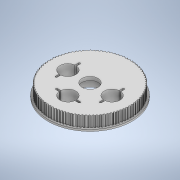
# Autodesk Inventor part: os_6_zebatka
Saved by Autodesk Inventor 2020.3 (Build 243373000, 373)
## iProperties
Created: 2021-03-12
Part Number: os_6_zebatka
Material: Generic
Document SubType Name: Modeling
Designer: patry
Density: 1 g/cm^3
Appearance: Default
Author: patry
Autodesk Inventor part; units mm, degrees
(part 1 of 2)
ref_plane "YZ Plane" through (0, 0, 0) normal (1, 0, 0) x (0, 1, 0)
ref_plane "XZ Plane" through (0, 0, 0) normal (0, 1, 0) x (-1, 0, 0)
ref_plane "XY Plane" through (0, 0, 0) normal (0, 0, 1) x (1, 0, 0)
sketch "Sketch1" plane through (0, 0, 0) normal (0, 1, 0) x (-1, 0, 0)
  circle A0 centre (0, 0) radius 47.5
  dimension "d0" = 95
  constraints: 1 centre point, 1 coincident
  measures "d0" diameter of A0
extrude "Extrusion1" add sketch "Sketch1" along normal blind 2
sketch "Sketch2" plane through (0, 2, 0) normal (0, 1, 0) x (1, 0, 0)
  circle A0 centre (0, 0) radius 45.5
  line L0 (0, 45.5) -> (0.3625, 45.5)
  line L1 (0.3625, 45.5) -> (-0.3625, 45.5)
  line L2 (-0.3625, 45.5) -> (0.3625, 45.5)
  arc A1 (-1.5, 44.3625) -> (-0.5625, 45.3) centre (-1.5, 45.3) ccw
  arc A2 (0.5625, 45.3) -> (1.5, 44.3625) centre (1.5, 45.3) ccw
  line L3 (-0.3625, 45.5) -> (0.3625, 45.5)
  arc A3 (-0.3625, 45.5) -> (-0.5625, 45.3) centre (-0.3625, 45.3) ccw
  arc A4 (0.5625, 45.3) -> (0.3625, 45.5) centre (0.3625, 45.3) ccw
  line L4 (-2.9452, 45.4046) -> (-2.5835, 45.428)
  line L5 (-2.5835, 45.428) -> (-3.3069, 45.3811)
  line L6 (-3.3069, 45.3811) -> (-2.5835, 45.428)
  arc A5 (-4.3684, 44.1724) -> (-3.4936, 45.1686) centre (-4.4291, 45.1079) ccw
  arc A6 (-2.3709, 45.2414) -> (-1.3747, 44.3666) centre (-1.4354, 45.3021) ccw
  line L7 (-3.3069, 45.3811) -> (-2.5835, 45.428)
  arc A7 (-3.3069, 45.3811) -> (-3.4936, 45.1686) centre (-3.294, 45.1815) ccw
  arc A8 (-2.3709, 45.2414) -> (-2.5835, 45.428) centre (-2.5705, 45.2285) ccw
  line L8 (-5.8781, 45.1187) -> (-5.5186, 45.1655)
  line L9 (-5.5186, 45.1655) -> (-6.2375, 45.0719)
  line L10 (-6.2375, 45.0719) -> (-5.5186, 45.1655)
  arc A9 (-7.2185, 43.797) -> (-6.41, 44.8477) centre (-7.3397, 44.7266) ccw
  arc A10 (-5.2944, 44.9931) -> (-4.2437, 44.1845) centre (-4.3648, 45.1142) ccw
  line L11 (-6.2375, 45.0719) -> (-5.5186, 45.1655)
  arc A11 (-6.2375, 45.0719) -> (-6.41, 44.8477) centre (-6.2117, 44.8736) ccw
  arc A12 (-5.2944, 44.9931) -> (-5.5186, 45.1655) centre (-5.4928, 44.9672) ccw
  line L12 (-8.7863, 44.6436) -> (-8.4306, 44.7136)
  line L13 (-8.4306, 44.7136) -> (-9.1419, 44.5736)
  line L14 (-9.1419, 44.5736) -> (-8.4306, 44.7136)
  arc A13 (-10.0384, 43.2379) -> (-9.2996, 44.3388) centre (-10.2194, 44.1577) ccw
  arc A14 (-8.1957, 44.556) -> (-7.0948, 43.8172) centre (-7.2759, 44.737) ccw
  line L15 (-9.1419, 44.5736) -> (-8.4306, 44.7136)
  arc A15 (-9.1419, 44.5736) -> (-9.2996, 44.3388) centre (-9.1033, 44.3774) ccw
  arc A16 (-8.1957, 44.556) -> (-8.4306, 44.7136) centre (-8.392, 44.5174) ccw
  line L16 (-11.6576, 43.9812) -> (-11.3072, 44.0741)
  line L17 (-11.3072, 44.0741) -> (-12.008, 43.8884)
  line L18 (-12.008, 43.8884) -> (-11.3072, 44.0741)
  arc A17 (-12.8161, 42.4974) -> (-12.1501, 43.6438) centre (-13.0563, 43.4036) ccw
  arc A18 (-11.0626, 43.932) -> (-9.9162, 43.266) centre (-10.1564, 44.1722) ccw
  line L19 (-12.008, 43.8884) -> (-11.3072, 44.0741)
  arc A19 (-12.008, 43.8884) -> (-12.1501, 43.6438) centre (-11.9568, 43.695) ccw
  arc A20 (-11.0626, 43.932) -> (-11.3072, 44.0741) centre (-11.256, 43.8808) ccw
  line L20 (-14.4801, 43.1344) -> (-14.1364, 43.2498)
  line L21 (-14.1364, 43.2498) -> (-14.8237, 43.0191)
  line L22 (-14.8237, 43.0191) -> (-14.1364, 43.2498)
  arc A21 (-15.5401, 41.5787) -> (-14.9497, 42.7658) centre (-15.8384, 42.4675) ccw
  arc A22 (-13.8832, 43.1238) -> (-12.696, 42.5334) centre (-12.9944, 43.4222) ccw
  line L23 (-14.8237, 43.0191) -> (-14.1364, 43.2498)
  arc A23 (-14.8237, 43.0191) -> (-14.9497, 42.7658) centre (-14.7601, 42.8295) ccw
  arc A24 (-13.8832, 43.1238) -> (-14.1364, 43.2498) centre (-14.0728, 43.0602) ccw
  line L24 (-17.2418, 42.1067) -> (-16.9063, 42.244)
  line L25 (-16.9063, 42.244) -> (-17.5772, 41.9693)
  line L26 (-17.5772, 41.9693) -> (-16.9063, 42.244)
  arc A25 (-18.1989, 40.4856) -> (-17.6865, 41.7084) centre (-18.5541, 41.3532) ccw
  arc A26 (-16.6454, 42.1347) -> (-15.4226, 41.6224) centre (-15.7779, 42.49) ccw
  line L27 (-17.5772, 41.9693) -> (-16.9063, 42.244)
  arc A27 (-17.5772, 41.9693) -> (-17.6865, 41.7084) centre (-17.5014, 41.7842) ccw
  arc A28 (-16.6454, 42.1347) -> (-16.9063, 42.244) centre (-16.8305, 42.0589) ccw
  line L28 (-19.9312, 40.9023) -> (-19.6053, 41.0611)
  line L29 (-19.6053, 41.0611) -> (-20.257, 40.7435)
  line L30 (-20.257, 40.7435) -> (-19.6053, 41.0611)
  arc A29 (-20.7813, 39.2227) -> (-20.3492, 40.4761) centre (-21.192, 40.0654) ccw
  arc A30 (-19.3379, 40.9689) -> (-18.0845, 40.5368) centre (-18.4951, 41.3796) ccw
  line L31 (-20.257, 40.7435) -> (-19.6053, 41.0611)
  arc A31 (-20.257, 40.7435) -> (-20.3492, 40.4761) centre (-20.1694, 40.5637) ccw
  arc A32 (-19.3379, 40.9689) -> (-19.6053, 41.0611) centre (-19.5177, 40.8813) ccw
  line L32 (-22.537, 39.5264) -> (-22.2221, 39.7059)
  line L33 (-22.2221, 39.7059) -> (-22.8519, 39.3468)
  line L34 (-22.8519, 39.3468) -> (-22.2221, 39.7059)
  arc A33 (-23.2766, 37.7952) -> (-22.9266, 39.074) centre (-23.741, 38.6097) ccw
  arc A34 (-21.9493, 39.6313) -> (-20.6705, 39.2812) centre (-21.1348, 40.0956) ccw
  line L35 (-22.8519, 39.3468) -> (-22.2221, 39.7059)
  arc A35 (-22.8519, 39.3468) -> (-22.9266, 39.074) centre (-22.7528, 39.1731) ccw
  arc A36 (-21.9493, 39.6313) -> (-22.2221, 39.7059) centre (-22.123, 39.5322) ccw
  line L36 (-25.0482, 37.9847) -> (-24.7456, 38.1842)
  line L37 (-24.7456, 38.1842) -> (-25.3509, 37.7851)
  line L38 (-25.3509, 37.7851) -> (-24.7456, 38.1842)
  arc A37 (-25.6743, 36.2093) -> (-25.4077, 37.508) centre (-26.1904, 36.9919) ccw
  arc A38 (-24.4685, 38.1274) -> (-23.1698, 37.8608) centre (-23.6859, 38.6435) ccw
  line L39 (-25.3509, 37.7851) -> (-24.7456, 38.1842)
  arc A39 (-25.3509, 37.7851) -> (-25.4077, 37.508) centre (-25.2408, 37.6182) ccw
  arc A40 (-24.4685, 38.1274) -> (-24.7456, 38.1842) centre (-24.6355, 38.0173) ccw
  line L40 (-27.4545, 36.2836) -> (-27.1654, 36.5024)
  line L41 (-27.1654, 36.5024) -> (-27.7435, 36.0649)
  line L42 (-27.7435, 36.0649) -> (-27.1654, 36.5024)
  arc A41 (-27.9643, 34.4715) -> (-27.7823, 35.7847) centre (-28.5299, 35.2191) ccw
  arc A42 (-26.8852, 36.4636) -> (-25.5719, 36.2816) centre (-26.1376, 37.0293) ccw
  line L43 (-27.7435, 36.0649) -> (-27.1654, 36.5024)
  arc A43 (-27.7435, 36.0649) -> (-27.7823, 35.7847) centre (-27.6228, 35.9054) ccw
  arc A44 (-26.8852, 36.4636) -> (-27.1654, 36.5024) centre (-27.0447, 36.3429) ccw
  line L44 (-29.7455, 34.4304) -> (-29.4712, 34.6674)
  line L45 (-29.4712, 34.6674) -> (-30.0198, 34.1934)
  line L46 (-30.0198, 34.1934) -> (-29.4712, 34.6674)
  arc A45 (-30.1369, 32.5891) -> (-30.0404, 33.9114) centre (-30.7498, 33.2985) ccw
  arc A46 (-29.1891, 34.6468) -> (-27.8668, 34.5503) centre (-28.4797, 35.2597) ccw
  line L47 (-30.0198, 34.1934) -> (-29.4712, 34.6674)
  arc A47 (-30.0198, 34.1934) -> (-30.0404, 33.9114) centre (-29.8891, 34.0421) ccw
  arc A48 (-29.1891, 34.6468) -> (-29.4712, 34.6674) centre (-29.3405, 34.5161) ccw
  line L48 (-31.9118, 32.4328) -> (-31.6534, 32.687)
  line L49 (-31.6534, 32.687) -> (-32.1702, 32.1786)
  line L50 (-32.1702, 32.1786) -> (-31.6534, 32.687)
  arc A49 (-32.1832, 30.5699) -> (-32.1725, 31.8957) centre (-32.8407, 31.2382) ccw
  arc A50 (-31.3706, 32.6848) -> (-30.0448, 32.674) centre (-30.7023, 33.3423) ccw
  line L51 (-32.1702, 32.1786) -> (-31.6534, 32.687)
  arc A51 (-32.1702, 32.1786) -> (-32.1725, 31.8957) centre (-32.0299, 32.036) ccw
  arc A52 (-31.3706, 32.6848) -> (-31.6534, 32.687) centre (-31.5131, 32.5445) ccw
  line L52 (-33.9442, 30.2991) -> (-33.7029, 30.5696)
  line L53 (-33.7029, 30.5696) -> (-34.1856, 30.0287)
  line L54 (-34.1856, 30.0287) -> (-33.7029, 30.5696)
  arc A53 (-34.0945, 28.4226) -> (-34.1696, 29.7463) centre (-34.7939, 29.0469) ccw
  arc A54 (-33.4205, 30.5856) -> (-32.0968, 30.6607) centre (-32.7962, 31.285) ccw
  line L55 (-34.1856, 30.0287) -> (-33.7029, 30.5696)
  arc A55 (-34.1856, 30.0287) -> (-34.1696, 29.7463) centre (-34.0364, 29.8955) ccw
  arc A56 (-33.4205, 30.5856) -> (-33.7029, 30.5696) centre (-33.5536, 30.4364) ccw
  line L56 (-35.8343, 28.0384) -> (-35.6109, 28.3239)
  line L57 (-35.6109, 28.3239) -> (-36.0577, 27.7529)
  line L58 (-36.0577, 27.7529) -> (-35.6109, 28.3239)
  arc A57 (-35.8628, 26.1561) -> (-36.0234, 27.4721) centre (-36.6011, 26.7338) ccw
  arc A58 (-35.3302, 28.3582) -> (-34.0141, 28.5188) centre (-34.7525, 29.0965) ccw
  line L59 (-36.0577, 27.7529) -> (-35.6109, 28.3239)
  arc A59 (-36.0577, 27.7529) -> (-36.0234, 27.4721) centre (-35.9002, 27.6297) ccw
  arc A60 (-35.3302, 28.3582) -> (-35.6109, 28.3239) centre (-35.4534, 28.2006) ccw
  line L60 (-37.5741, 25.66) -> (-37.3697, 25.9594)
  line L61 (-37.3697, 25.9594) -> (-37.7785, 25.3607)
  line L62 (-37.7785, 25.3607) -> (-37.3697, 25.9594)
  arc A61 (-37.4807, 23.7798) -> (-37.7262, 25.0827) centre (-38.2549, 24.3085) ccw
  arc A62 (-37.0917, 26.0118) -> (-35.7888, 26.2572) centre (-36.563, 26.786) ccw
  line L63 (-37.7785, 25.3607) -> (-37.3697, 25.9594)
  arc A63 (-37.7785, 25.3607) -> (-37.7262, 25.0827) centre (-37.6134, 25.2479) ccw
  arc A64 (-37.0917, 26.0118) -> (-37.3697, 25.9594) centre (-37.2045, 25.8466) ccw
  line L64 (-39.1563, 23.1741) -> (-38.9716, 23.486)
  line L65 (-38.9716, 23.486) -> (-39.3409, 22.8621)
  line L66 (-39.3409, 22.8621) -> (-38.9716, 23.486)
  arc A65 (-38.9413, 21.3039) -> (-39.2706, 22.5881) centre (-39.7481, 21.7813) ccw
  arc A66 (-38.6977, 23.5563) -> (-37.4134, 23.8856) centre (-38.2202, 24.3631) ccw
  line L67 (-39.3409, 22.8621) -> (-38.9716, 23.486)
  arc A67 (-39.3409, 22.8621) -> (-39.2706, 22.5881) centre (-39.1688, 22.7602) ccw
  arc A68 (-38.6977, 23.5563) -> (-38.9716, 23.486) centre (-38.7995, 23.3842) ccw
  line L68 (-40.5742, 20.5909) -> (-40.4101, 20.9141)
  line L69 (-40.4101, 20.9141) -> (-40.7382, 20.2676)
  line L70 (-40.7382, 20.2676) -> (-40.4101, 20.9141)
  arc A69 (-40.2387, 18.7385) -> (-40.6504, 19.9988) centre (-41.0747, 19.1628) ccw
  arc A70 (-40.1413, 21.002) -> (-38.881, 21.4137) centre (-39.717, 21.838) ccw
  line L71 (-40.7382, 20.2676) -> (-40.4101, 20.9141)
  arc A71 (-40.7382, 20.2676) -> (-40.6504, 19.9988) centre (-40.5599, 20.1771) ccw
  arc A72 (-40.1413, 21.002) -> (-40.4101, 20.9141) centre (-40.2318, 20.8236) ccw
  line L72 (-41.8219, 17.9213) -> (-41.6792, 18.2545)
  line L73 (-41.6792, 18.2545) -> (-41.9647, 17.5882)
  line L74 (-41.9647, 17.5882) -> (-41.6792, 18.2545)
  arc A73 (-41.3672, 16.0946) -> (-41.8597, 17.3255) centre (-42.2289, 16.4638) ccw
  arc A74 (-41.4166, 18.3596) -> (-40.1856, 18.8521) centre (-41.0473, 19.2213) ccw
  line L75 (-41.9647, 17.5882) -> (-41.6792, 18.2545)
  arc A75 (-41.9647, 17.5882) -> (-41.8597, 17.3255) centre (-41.7809, 17.5094) ccw
  arc A76 (-41.4166, 18.3596) -> (-41.6792, 18.2545) centre (-41.4953, 18.1758) ccw
  line L76 (-42.8943, 15.1766) -> (-42.7734, 15.5184)
  line L77 (-42.7734, 15.5184) -> (-43.0152, 14.8349)
  line L78 (-43.0152, 14.8349) -> (-42.7734, 15.5184)
  arc A77 (-42.3223, 13.3831) -> (-42.8934, 14.5796) centre (-43.2061, 13.6958) ccw
  arc A78 (-42.5181, 15.6402) -> (-41.3216, 16.2113) centre (-42.2054, 16.524) ccw
  line L79 (-43.0152, 14.8349) -> (-42.7734, 15.5184)
  arc A79 (-43.0152, 14.8349) -> (-42.8934, 14.5796) centre (-42.8267, 14.7682) ccw
  arc A80 (-42.5181, 15.6402) -> (-42.7734, 15.5184) centre (-42.5848, 15.4517) ccw
  line L80 (-43.7867, 12.3683) -> (-43.6882, 12.7171)
  line L81 (-43.6882, 12.7171) -> (-43.8852, 12.0194)
  line L82 (-43.8852, 12.0194) -> (-43.6882, 12.7171)
  arc A81 (-43.0998, 10.6155) -> (-43.7471, 11.7726) centre (-44.002, 10.8704) ccw
  arc A82 (-43.4413, 12.8552) -> (-42.2843, 13.5026) centre (-43.1865, 13.7574) ccw
  line L83 (-43.8852, 12.0194) -> (-43.6882, 12.7171)
  arc A83 (-43.8852, 12.0194) -> (-43.7471, 11.7726) centre (-43.6928, 11.9651) ccw
  arc A84 (-43.4413, 12.8552) -> (-43.6882, 12.7171) centre (-43.4957, 12.6628) ccw
  line L84 (-44.4955, 9.508) -> (-44.4197, 9.8625)
  line L85 (-44.4197, 9.8625) -> (-44.5712, 9.1535)
  line L86 (-44.5712, 9.1535) -> (-44.4197, 9.8625)
  arc A85 (-43.6965, 7.8034) -> (-44.4174, 8.9161) centre (-44.6133, 7.9993) ccw
  arc A86 (-44.1823, 10.0163) -> (-43.0696, 10.7372) centre (-43.9864, 10.9331) ccw
  line L87 (-44.5712, 9.1535) -> (-44.4197, 9.8625)
  arc A87 (-44.5712, 9.1535) -> (-44.4174, 8.9161) centre (-44.3756, 9.1117) ccw
  arc A88 (-44.1823, 10.0163) -> (-44.4197, 9.8625) centre (-44.2241, 9.8207) ccw
  line L88 (-45.0176, 6.6079) -> (-44.965, 6.9666)
  line L89 (-44.965, 6.9666) -> (-45.0703, 6.2492)
  line L90 (-45.0703, 6.2492) -> (-44.965, 6.9666)
  arc A89 (-44.11, 4.9586) -> (-44.9014, 6.0223) centre (-45.0376, 5.0948) ccw
  arc A90 (-44.738, 7.1354) -> (-43.6743, 7.9268) centre (-44.6019, 8.063) ccw
  line L91 (-45.0703, 6.2492) -> (-44.965, 6.9666)
  arc A91 (-45.0703, 6.2492) -> (-44.9014, 6.0223) centre (-44.8724, 6.2202) ccw
  arc A92 (-44.738, 7.1354) -> (-44.965, 6.9666) centre (-44.7671, 6.9375) ccw
  line L92 (-45.3509, 3.6801) -> (-45.3216, 4.0414)
  line L93 (-45.3216, 4.0414) -> (-45.3803, 3.3187)
  line L94 (-45.3803, 3.3187) -> (-45.3216, 4.0414)
  arc A93 (-44.3385, 2.093) -> (-45.1971, 3.1032) centre (-45.2729, 2.1688) ccw
  arc A94 (-45.1061, 4.2245) -> (-44.0958, 5.0831) centre (-45.0303, 5.159) ccw
  line L95 (-45.3803, 3.3187) -> (-45.3216, 4.0414)
  arc A95 (-45.3803, 3.3187) -> (-45.1971, 3.1032) centre (-45.1809, 3.3026) ccw
  arc A96 (-45.1061, 4.2245) -> (-45.3216, 4.0414) centre (-45.1223, 4.0252) ccw
  line L96 (-45.494, 0.7368) -> (-45.4882, 1.0992)
  line L97 (-45.4882, 1.0992) -> (-45.4999, 0.3743)
  line L98 (-45.4999, 0.3743) -> (-45.4882, 1.0992)
  arc A97 (-44.381, -0.7814) -> (-45.3032, 0.1711) centre (-45.3184, -0.7663) ccw
  arc A98 (-45.285, 1.296) -> (-44.3324, 2.2182) centre (-45.2698, 2.2333) ccw
  line L99 (-45.4999, 0.3743) -> (-45.4882, 1.0992)
  arc A99 (-45.4999, 0.3743) -> (-45.3032, 0.1711) centre (-45.2999, 0.3711) ccw
  arc A100 (-45.285, 1.296) -> (-45.4882, 1.0992) centre (-45.2882, 1.096) ccw
  line L100 (-45.4463, -2.2096) -> (-45.4639, -1.8475)
  line L101 (-45.4639, -1.8475) -> (-45.4287, -2.5717)
  line L102 (-45.4287, -2.5717) -> (-45.4639, -1.8475)
  arc A101 (-44.2373, -3.6526) -> (-45.2192, -2.7617) centre (-45.1737, -3.6981) ccw
  arc A102 (-45.2739, -1.638) -> (-44.383, -0.6561) centre (-45.3194, -0.7016) ccw
  line L103 (-45.4287, -2.5717) -> (-45.4639, -1.8475)
  arc A103 (-45.4287, -2.5717) -> (-45.2192, -2.7617) centre (-45.2289, -2.5619) ccw
  arc A104 (-45.2739, -1.638) -> (-45.4639, -1.8475) centre (-45.2642, -1.8378) ccw
  line L104 (-45.208, -5.1467) -> (-45.249, -4.7865)
  line L105 (-45.249, -4.7865) -> (-45.167, -5.5069)
  line L106 (-45.167, -5.5069) -> (-45.249, -4.7865)
  arc A105 (-43.9081, -6.5084) -> (-44.9456, -5.6829) centre (-44.8396, -6.6144) ccw
  arc A106 (-45.0729, -4.5652) -> (-44.2475, -3.5276) centre (-45.1789, -3.6337) ccw
  line L107 (-45.167, -5.5069) -> (-45.249, -4.7865)
  arc A107 (-45.167, -5.5069) -> (-44.9456, -5.6829) centre (-44.9683, -5.4842) ccw
  arc A108 (-45.0729, -4.5652) -> (-45.249, -4.7865) centre (-45.0503, -4.7639) ccw
  line L108 (-44.78, -8.0622) -> (-44.8443, -7.7054)
  line L109 (-44.8443, -7.7054) -> (-44.7158, -8.419)
  line L110 (-44.7158, -8.419) -> (-44.8443, -7.7054)
  arc A109 (-43.3947, -9.3369) -> (-44.4835, -8.5804) centre (-44.3174, -9.503) ccw
  arc A110 (-44.6829, -7.4732) -> (-43.9263, -6.3844) centre (-44.849, -6.5505) ccw
  line L111 (-44.7158, -8.419) -> (-44.8443, -7.7054)
  arc A111 (-44.7158, -8.419) -> (-44.4835, -8.5804) centre (-44.519, -8.3835) ccw
  arc A112 (-44.6829, -7.4732) -> (-44.8443, -7.7054) centre (-44.6474, -7.67) ccw
  line L112 (-44.1643, -10.9439) -> (-44.2514, -10.592)
  line L113 (-44.2514, -10.592) -> (-44.0771, -11.2957)
  line L114 (-44.0771, -11.2957) -> (-44.2514, -10.592)
  arc A113 (-42.6994, -12.1263) -> (-43.8348, -11.4418) centre (-43.6093, -12.3517) ccw
  arc A114 (-44.1054, -10.3498) -> (-43.4209, -9.2143) centre (-44.3309, -9.4398) ccw
  line L115 (-44.0771, -11.2957) -> (-44.2514, -10.592)
  arc A115 (-44.0771, -11.2957) -> (-43.8348, -11.4418) centre (-43.8829, -11.2476) ccw
  arc A116 (-44.1054, -10.3498) -> (-44.2514, -10.592) centre (-44.0573, -10.5439) ccw
  line L116 (-43.3632, -13.7797) -> (-43.473, -13.4342)
  line L117 (-43.473, -13.4342) -> (-43.2535, -14.1252)
  line L118 (-43.2535, -14.1252) -> (-43.473, -13.4342)
  arc A117 (-41.8249, -14.8647) -> (-43.0023, -14.2552) centre (-42.7184, -15.1487) ccw
  arc A118 (-43.343, -13.183) -> (-42.7334, -12.0056) centre (-43.6269, -12.2896) ccw
  line L119 (-43.2535, -14.1252) -> (-43.473, -13.4342)
  arc A119 (-43.2535, -14.1252) -> (-43.0023, -14.2552) centre (-43.0628, -14.0646) ccw
  arc A120 (-43.343, -13.183) -> (-43.473, -13.4342) centre (-43.2824, -13.3736) ccw
  line L120 (-42.3803, -16.5577) -> (-42.5123, -16.22)
  line L121 (-42.5123, -16.22) -> (-42.2484, -16.8953)
  line L122 (-42.2484, -16.8953) -> (-42.5123, -16.22)
  arc A121 (-40.775, -17.5409) -> (-41.9894, -17.0088) centre (-41.6482, -17.882) ccw
  arc A122 (-42.3988, -15.961) -> (-41.8667, -14.7466) centre (-42.7399, -15.0877) ccw
  line L123 (-42.2484, -16.8953) -> (-42.5123, -16.22)
  arc A123 (-42.2484, -16.8953) -> (-41.9894, -17.0088) centre (-42.0621, -16.8225) ccw
  arc A124 (-42.3988, -15.961) -> (-42.5123, -16.22) centre (-42.326, -16.1472) ccw
  line L124 (-41.2197, -19.2662) -> (-41.3732, -18.9378)
  line L125 (-41.3732, -18.9378) -> (-41.0662, -19.5946)
  line L126 (-41.0662, -19.5946) -> (-41.3732, -18.9378)
  arc A125 (-39.554, -20.1435) -> (-40.8003, -19.6911) centre (-40.4034, -20.5404) ccw
  arc A126 (-41.2767, -18.672) -> (-40.8243, -17.4257) centre (-41.6737, -17.8226) ccw
  line L127 (-41.0662, -19.5946) -> (-41.3732, -18.9378)
  arc A127 (-41.0662, -19.5946) -> (-40.8003, -19.6911) centre (-40.885, -19.5099) ccw
  arc A128 (-41.2767, -18.672) -> (-41.3732, -18.9378) centre (-41.192, -18.8531) ccw
  line L128 (-39.8861, -21.894) -> (-40.0606, -21.5762)
  line L129 (-40.0606, -21.5762) -> (-39.7117, -22.2117)
  line L130 (-39.7117, -22.2117) -> (-40.0606, -21.5762)
  arc A129 (-38.1672, -22.6615) -> (-39.4402, -22.2908) centre (-38.989, -23.1127) ccw
  arc A130 (-39.9815, -21.3046) -> (-39.6108, -20.0317) centre (-40.4326, -20.4828) ccw
  line L131 (-39.7117, -22.2117) -> (-40.0606, -21.5762)
  arc A131 (-39.7117, -22.2117) -> (-39.4402, -22.2908) centre (-39.5364, -22.1155) ccw
  arc A132 (-39.9815, -21.3046) -> (-40.0606, -21.5762) centre (-39.8853, -21.4799) ccw
  line L132 (-38.3853, -24.4299) -> (-38.5799, -24.1241)
  line L133 (-38.5799, -24.1241) -> (-38.1907, -24.7357)
  line L134 (-38.1907, -24.7357) -> (-38.5799, -24.1241)
  arc A133 (-36.6203, -25.0846) -> (-37.9146, -24.797) centre (-37.4112, -25.5879) ccw
  arc A134 (-38.5186, -23.8479) -> (-38.2311, -22.5537) centre (-39.022, -23.057) ccw
  line L135 (-38.1907, -24.7357) -> (-38.5799, -24.1241)
  arc A135 (-38.1907, -24.7357) -> (-37.9146, -24.797) centre (-38.0219, -24.6283) ccw
  arc A136 (-38.5186, -23.8479) -> (-38.5799, -24.1241) centre (-38.4112, -24.0167) ccw
  line L136 (-36.7235, -26.8633) -> (-36.9375, -26.5707)
  line L137 (-36.9375, -26.5707) -> (-36.5094, -27.1559)
  line L138 (-36.5094, -27.1559) -> (-36.9375, -26.5707)
  arc A137 (-34.9198, -27.4024) -> (-36.2299, -27.1992) centre (-35.6764, -27.9559) ccw
  arc A138 (-36.8941, -26.2912) -> (-36.691, -24.9811) centre (-37.4476, -25.5346) ccw
  line L139 (-36.5094, -27.1559) -> (-36.9375, -26.5707)
  arc A139 (-36.5094, -27.1559) -> (-36.2299, -27.1992) centre (-36.348, -27.0378) ccw
  arc A140 (-36.8941, -26.2912) -> (-36.9375, -26.5707) centre (-36.7761, -26.4527) ccw
  line L140 (-34.9076, -29.1841) -> (-35.1401, -28.906)
  line L141 (-35.1401, -28.906) -> (-34.6751, -29.4622)
  line L142 (-34.6751, -29.4622) -> (-35.1401, -28.906)
  arc A141 (-33.0728, -29.6053) -> (-34.3934, -29.4873) centre (-33.792, -30.2066) ccw
  arc A142 (-35.1149, -28.6242) -> (-34.997, -27.3037) centre (-35.7163, -27.905) ccw
  line L143 (-34.6751, -29.4622) -> (-35.1401, -28.906)
  arc A143 (-34.6751, -29.4622) -> (-34.3934, -29.4873) centre (-34.5216, -29.3339) ccw
  arc A144 (-35.1149, -28.6242) -> (-35.1401, -28.906) centre (-34.9867, -28.7777) ccw
  line L144 (-32.9453, -31.3824) -> (-33.1953, -31.12)
  line L145 (-33.1953, -31.12) -> (-32.6953, -31.6449)
  line L146 (-32.6953, -31.6449) -> (-33.1953, -31.12)
  arc A145 (-31.0871, -31.684) -> (-32.4125, -31.6518) centre (-31.7659, -32.3306) ccw
  arc A146 (-33.1885, -30.8372) -> (-33.1563, -29.5118) centre (-33.8351, -30.1584) ccw
  line L147 (-32.6953, -31.6449) -> (-33.1953, -31.12)
  arc A147 (-32.6953, -31.6449) -> (-32.4125, -31.6518) centre (-32.5505, -31.507) ccw
  arc A148 (-33.1885, -30.8372) -> (-33.1953, -31.12) centre (-33.0505, -30.982) ccw
  line L148 (-30.8448, -33.4492) -> (-31.1113, -33.2034)
  line L149 (-31.1113, -33.2034) -> (-30.5783, -33.6949)
  line L150 (-30.5783, -33.6949) -> (-31.1113, -33.2034)
  arc A149 (-28.971, -33.6298) -> (-30.2957, -33.6835) centre (-29.6065, -34.319) ccw
  arc A150 (-31.1228, -32.9208) -> (-31.1764, -31.5961) centre (-31.812, -32.2853) ccw
  line L151 (-30.5783, -33.6949) -> (-31.1113, -33.2034)
  arc A151 (-30.5783, -33.6949) -> (-30.2957, -33.6835) centre (-30.4428, -33.5479) ccw
  arc A152 (-31.1228, -32.9208) -> (-31.1113, -33.2034) centre (-30.9757, -33.0564) ccw
  line L152 (-28.615, -35.3756) -> (-28.8968, -35.1476)
  line L153 (-28.8968, -35.1476) -> (-28.3331, -35.6036)
  line L154 (-28.3331, -35.6036) -> (-28.8968, -35.1476)
  arc A153 (-26.7334, -35.4346) -> (-28.0519, -35.5739) centre (-27.323, -36.1634) ccw
  arc A154 (-28.9265, -34.8663) -> (-29.0658, -33.5479) centre (-29.6554, -34.2767) ccw
  line L155 (-28.3331, -35.6036) -> (-28.8968, -35.1476)
  arc A155 (-28.3331, -35.6036) -> (-28.0519, -35.5739) centre (-28.2074, -35.4481) ccw
  arc A156 (-28.9265, -34.8663) -> (-28.8968, -35.1476) centre (-28.771, -34.9921) ccw
  line L156 (-26.2651, -37.1536) -> (-26.5611, -36.9444)
  line L157 (-26.5611, -36.9444) -> (-25.9691, -37.3629)
  line L158 (-25.9691, -37.3629) -> (-26.5611, -36.9444)
  arc A157 (-24.3836, -37.0907) -> (-25.6904, -37.315) centre (-24.9248, -37.8562) ccw
  arc A158 (-26.609, -36.6656) -> (-26.8333, -35.3589) centre (-27.3745, -36.1245) ccw
  line L159 (-25.9691, -37.3629) -> (-26.5611, -36.9444)
  arc A159 (-25.9691, -37.3629) -> (-25.6904, -37.315) centre (-25.8537, -37.1996) ccw
  arc A160 (-26.609, -36.6656) -> (-26.5611, -36.9444) centre (-26.4457, -36.7811) ccw
  line L160 (-23.8051, -38.7759) -> (-24.114, -38.5862)
  line L161 (-24.114, -38.5862) -> (-23.4962, -38.9655)
  line L162 (-23.4962, -38.9655) -> (-24.114, -38.5862)
  arc A161 (-21.9316, -38.5913) -> (-23.2211, -38.8997) centre (-22.4221, -39.3902) ccw
  arc A162 (-24.1798, -38.3111) -> (-24.4883, -37.0217) centre (-24.9788, -37.8206) ccw
  line L163 (-23.4962, -38.9655) -> (-24.114, -38.5862)
  arc A163 (-23.4962, -38.9655) -> (-23.2211, -38.8997) centre (-23.3915, -38.7951) ccw
  arc A164 (-24.1798, -38.3111) -> (-24.114, -38.5862) centre (-24.0094, -38.4158) ccw
  line L164 (-21.2452, -40.2354) -> (-21.5658, -40.0662)
  line L165 (-21.5658, -40.0662) -> (-20.9247, -40.4047)
  line L166 (-20.9247, -40.4047) -> (-21.5658, -40.0662)
  arc A165 (-19.3876, -39.93) -> (-20.6544, -40.3212) centre (-19.8254, -40.759) ccw
  arc A166 (-21.6492, -39.7959) -> (-22.0405, -38.5292) centre (-22.4783, -39.3582) ccw
  line L167 (-20.9247, -40.4047) -> (-21.5658, -40.0662)
  arc A167 (-20.9247, -40.4047) -> (-20.6544, -40.3212) centre (-20.8313, -40.2278) ccw
  arc A168 (-21.6492, -39.7959) -> (-21.5658, -40.0662) centre (-21.4724, -39.8893) ccw
  line L168 (-18.5962, -41.5263) -> (-18.9271, -41.3781)
  line L169 (-18.9271, -41.3781) -> (-18.2654, -41.6744)
  line L170 (-18.2654, -41.6744) -> (-18.9271, -41.3781)
  arc A169 (-16.7623, -41.1012) -> (-18.0011, -41.5736) centre (-17.1455, -41.9568) ccw
  arc A170 (-19.0279, -41.1138) -> (-19.5003, -39.875) centre (-19.8835, -40.7307) ccw
  line L171 (-18.2654, -41.6744) -> (-18.9271, -41.3781)
  arc A171 (-18.2654, -41.6744) -> (-18.0011, -41.5736) centre (-18.1836, -41.4919) ccw
  arc A172 (-19.0279, -41.1138) -> (-18.9271, -41.3781) centre (-18.8453, -41.1956) ccw
  line L172 (-15.8692, -42.6429) -> (-16.209, -42.5165)
  line L173 (-16.209, -42.5165) -> (-15.5295, -42.7693)
  line L174 (-15.5295, -42.7693) -> (-16.209, -42.5165)
  arc A173 (-14.0667, -42.1) -> (-15.2723, -42.6516) centre (-14.3937, -42.9786) ccw
  arc A174 (-16.3267, -42.2593) -> (-16.8783, -41.0537) centre (-17.2053, -41.9323) ccw
  line L175 (-15.5295, -42.7693) -> (-16.209, -42.5165)
  arc A175 (-15.5295, -42.7693) -> (-15.2723, -42.6516) centre (-15.4597, -42.5819) ccw
  arc A176 (-16.3267, -42.2593) -> (-16.209, -42.5165) centre (-16.1392, -42.329) ccw
  line L176 (-13.0757, -43.5807) -> (-13.4229, -43.4765)
  line L177 (-13.4229, -43.4765) -> (-12.7285, -43.6849)
  line L178 (-12.7285, -43.6849) -> (-13.4229, -43.4765)
  arc A177 (-11.3121, -42.9222) -> (-12.4794, -43.5508) centre (-11.5815, -43.8202) ccw
  arc A178 (-13.557, -43.2275) -> (-14.1855, -42.0601) centre (-14.4549, -42.9581) ccw
  line L179 (-12.7285, -43.6849) -> (-13.4229, -43.4765)
  arc A179 (-12.7285, -43.6849) -> (-12.4794, -43.5508) centre (-12.671, -43.4933) ccw
  arc A180 (-13.557, -43.2275) -> (-13.4229, -43.4765) centre (-13.3654, -43.285) ccw
  line L180 (-10.2273, -44.3357) -> (-10.5805, -44.2542)
  line L181 (-10.5805, -44.2542) -> (-9.8741, -44.4172)
  line L182 (-9.8741, -44.4172) -> (-10.5805, -44.2542)
  arc A181 (-8.51, -43.5645) -> (-9.6342, -44.2672) centre (-8.7207, -44.478) ccw
  arc A182 (-10.7304, -44.0144) -> (-11.4332, -42.8901) centre (-11.644, -43.8036) ccw
  line L183 (-9.8741, -44.4172) -> (-10.5805, -44.2542)
  arc A183 (-9.8741, -44.4172) -> (-9.6342, -44.2672) centre (-9.8291, -44.2223) ccw
  arc A184 (-10.7304, -44.0144) -> (-10.5805, -44.2542) centre (-10.5356, -44.0593) ccw
  line L184 (-7.336, -44.9047) -> (-7.6938, -44.8463)
  line L185 (-7.6938, -44.8463) -> (-6.9782, -44.9632)
  line L186 (-6.9782, -44.9632) -> (-7.6938, -44.8463)
  arc A185 (-5.6722, -44.0239) -> (-6.7486, -44.798) centre (-5.8234, -44.9492) ccw
  arc A186 (-7.8589, -44.6166) -> (-8.633, -43.5402) centre (-8.7841, -44.4655) ccw
  line L187 (-6.9782, -44.9632) -> (-7.6938, -44.8463)
  arc A187 (-6.9782, -44.9632) -> (-6.7486, -44.798) centre (-6.946, -44.7658) ccw
  arc A188 (-7.8589, -44.6166) -> (-7.6938, -44.8463) centre (-7.6615, -44.6489) ccw
  line L188 (-4.4139, -45.2854) -> (-4.7747, -45.2502)
  line L189 (-4.7747, -45.2502) -> (-4.0532, -45.3206)
  line L190 (-4.0532, -45.3206) -> (-4.7747, -45.2502)
  arc A189 (-2.8107, -44.2988) -> (-3.8347, -45.1409) centre (-2.9016, -45.2319) ccw
  arc A190 (-4.9544, -45.0318) -> (-5.7965, -44.0077) centre (-5.8875, -44.9408) ccw
  line L191 (-4.0532, -45.3206) -> (-4.7747, -45.2502)
  arc A191 (-4.0532, -45.3206) -> (-3.8347, -45.1409) centre (-4.0338, -45.1215) ccw
  arc A192 (-4.9544, -45.0318) -> (-4.7747, -45.2502) centre (-4.7553, -45.0512) ccw
  line L192 (-1.4734, -45.4761) -> (-1.8357, -45.4644)
  line L193 (-1.8357, -45.4644) -> (-1.1111, -45.4879)
  line L194 (-1.1111, -45.4879) -> (-1.8357, -45.4644)
  arc A193 (0.0627, -44.3878) -> (-0.9047, -45.2945) centre (0.0323, -45.3248) ccw
  arc A194 (-2.0291, -45.258) -> (-2.9358, -44.2907) centre (-2.9661, -45.2277) ccw
  line L195 (-1.1111, -45.4879) -> (-1.8357, -45.4644)
  arc A195 (-1.1111, -45.4879) -> (-0.9047, -45.2945) centre (-1.1046, -45.288) ccw
  arc A196 (-2.0291, -45.258) -> (-1.8357, -45.4644) centre (-1.8292, -45.2645) ccw
  line L196 (1.4734, -45.4761) -> (1.1111, -45.4879)
  line L197 (1.1111, -45.4879) -> (1.8357, -45.4644)
  line L198 (1.8357, -45.4644) -> (1.1111, -45.4879)
  arc A197 (2.9358, -44.2907) -> (2.0291, -45.258) centre (2.9661, -45.2277) ccw
  arc A198 (0.9047, -45.2945) -> (-0.0627, -44.3878) centre (-0.0323, -45.3248) ccw
  line L199 (1.8357, -45.4644) -> (1.1111, -45.4879)
  arc A199 (1.8357, -45.4644) -> (2.0291, -45.258) centre (1.8292, -45.2645) ccw
  arc A200 (0.9047, -45.2945) -> (1.1111, -45.4879) centre (1.1046, -45.288) ccw
  line L200 (4.4139, -45.2854) -> (4.0532, -45.3206)
  line L201 (4.0532, -45.3206) -> (4.7747, -45.2502)
  line L202 (4.7747, -45.2502) -> (4.0532, -45.3206)
  arc A201 (5.7965, -44.0077) -> (4.9544, -45.0318) centre (5.8875, -44.9408) ccw
  arc A202 (3.8347, -45.1409) -> (2.8107, -44.2988) centre (2.9016, -45.2319) ccw
  line L203 (4.7747, -45.2502) -> (4.0532, -45.3206)
  arc A203 (4.7747, -45.2502) -> (4.9544, -45.0318) centre (4.7553, -45.0512) ccw
  arc A204 (3.8347, -45.1409) -> (4.0532, -45.3206) centre (4.0338, -45.1215) ccw
  line L204 (7.336, -44.9047) -> (6.9782, -44.9632)
  line L205 (6.9782, -44.9632) -> (7.6938, -44.8463)
  line L206 (7.6938, -44.8463) -> (6.9782, -44.9632)
  arc A205 (8.633, -43.5402) -> (7.8589, -44.6166) centre (8.7841, -44.4655) ccw
  arc A206 (6.7486, -44.798) -> (5.6722, -44.0239) centre (5.8234, -44.9492) ccw
  line L207 (7.6938, -44.8463) -> (6.9782, -44.9632)
  arc A207 (7.6938, -44.8463) -> (7.8589, -44.6166) centre (7.6615, -44.6489) ccw
  arc A208 (6.7486, -44.798) -> (6.9782, -44.9632) centre (6.946, -44.7658) ccw
  line L208 (10.2273, -44.3357) -> (9.8741, -44.4172)
  line L209 (9.8741, -44.4172) -> (10.5805, -44.2542)
  line L210 (10.5805, -44.2542) -> (9.8741, -44.4172)
  arc A209 (11.4332, -42.8901) -> (10.7304, -44.0144) centre (11.644, -43.8036) ccw
  arc A210 (9.6342, -44.2672) -> (8.51, -43.5645) centre (8.7207, -44.478) ccw
  line L211 (10.5805, -44.2542) -> (9.8741, -44.4172)
  arc A211 (10.5805, -44.2542) -> (10.7304, -44.0144) centre (10.5356, -44.0593) ccw
  arc A212 (9.6342, -44.2672) -> (9.8741, -44.4172) centre (9.8291, -44.2223) ccw
  line L212 (13.0757, -43.5807) -> (12.7285, -43.6849)
  line L213 (12.7285, -43.6849) -> (13.4229, -43.4765)
  line L214 (13.4229, -43.4765) -> (12.7285, -43.6849)
  arc A213 (14.1855, -42.0601) -> (13.557, -43.2275) centre (14.4549, -42.9581) ccw
  arc A214 (12.4794, -43.5508) -> (11.3121, -42.9222) centre (11.5815, -43.8202) ccw
  line L215 (13.4229, -43.4765) -> (12.7285, -43.6849)
  arc A215 (13.4229, -43.4765) -> (13.557, -43.2275) centre (13.3654, -43.285) ccw
  arc A216 (12.4794, -43.5508) -> (12.7285, -43.6849) centre (12.671, -43.4933) ccw
  line L216 (15.8692, -42.6429) -> (15.5295, -42.7693)
  line L217 (15.5295, -42.7693) -> (16.209, -42.5165)
  line L218 (16.209, -42.5165) -> (15.5295, -42.7693)
  arc A217 (16.8783, -41.0537) -> (16.3267, -42.2593) centre (17.2053, -41.9323) ccw
  arc A218 (15.2723, -42.6516) -> (14.0667, -42.1) centre (14.3937, -42.9786) ccw
  line L219 (16.209, -42.5165) -> (15.5295, -42.7693)
  arc A219 (16.209, -42.5165) -> (16.3267, -42.2593) centre (16.1392, -42.329) ccw
  arc A220 (15.2723, -42.6516) -> (15.5295, -42.7693) centre (15.4597, -42.5819) ccw
  line L220 (18.5962, -41.5263) -> (18.2654, -41.6744)
  line L221 (18.2654, -41.6744) -> (18.9271, -41.3781)
  line L222 (18.9271, -41.3781) -> (18.2654, -41.6744)
  arc A221 (19.5003, -39.875) -> (19.0279, -41.1138) centre (19.8835, -40.7307) ccw
  arc A222 (18.0011, -41.5736) -> (16.7623, -41.1012) centre (17.1455, -41.9568) ccw
  line L223 (18.9271, -41.3781) -> (18.2654, -41.6744)
  arc A223 (18.9271, -41.3781) -> (19.0279, -41.1138) centre (18.8453, -41.1956) ccw
  arc A224 (18.0011, -41.5736) -> (18.2654, -41.6744) centre (18.1836, -41.4919) ccw
  line L224 (21.2452, -40.2354) -> (20.9247, -40.4047)
  line L225 (20.9247, -40.4047) -> (21.5658, -40.0662)
  line L226 (21.5658, -40.0662) -> (20.9247, -40.4047)
  arc A225 (22.0405, -38.5292) -> (21.6492, -39.7959) centre (22.4783, -39.3582) ccw
  arc A226 (20.6544, -40.3212) -> (19.3876, -39.93) centre (19.8254, -40.759) ccw
  line L227 (21.5658, -40.0662) -> (20.9247, -40.4047)
  arc A227 (21.5658, -40.0662) -> (21.6492, -39.7959) centre (21.4724, -39.8893) ccw
  arc A228 (20.6544, -40.3212) -> (20.9247, -40.4047) centre (20.8313, -40.2278) ccw
  line L228 (23.8051, -38.7759) -> (23.4962, -38.9655)
  line L229 (23.4962, -38.9655) -> (24.114, -38.5862)
  line L230 (24.114, -38.5862) -> (23.4962, -38.9655)
  arc A229 (24.4883, -37.0217) -> (24.1798, -38.3111) centre (24.9788, -37.8206) ccw
  arc A230 (23.2211, -38.8997) -> (21.9316, -38.5913) centre (22.4221, -39.3902) ccw
  line L231 (24.114, -38.5862) -> (23.4962, -38.9655)
  arc A231 (24.114, -38.5862) -> (24.1798, -38.3111) centre (24.0094, -38.4158) ccw
  arc A232 (23.2211, -38.8997) -> (23.4962, -38.9655) centre (23.3915, -38.7951) ccw
  line L232 (26.2651, -37.1536) -> (25.9691, -37.3629)
  line L233 (25.9691, -37.3629) -> (26.5611, -36.9444)
  line L234 (26.5611, -36.9444) -> (25.9691, -37.3629)
  arc A233 (26.8333, -35.3589) -> (26.609, -36.6656) centre (27.3745, -36.1245) ccw
  arc A234 (25.6904, -37.315) -> (24.3836, -37.0907) centre (24.9248, -37.8562) ccw
  line L235 (26.5611, -36.9444) -> (25.9691, -37.3629)
  arc A235 (26.5611, -36.9444) -> (26.609, -36.6656) centre (26.4457, -36.7811) ccw
  arc A236 (25.6904, -37.315) -> (25.9691, -37.3629) centre (25.8537, -37.1996) ccw
  line L236 (28.615, -35.3756) -> (28.3331, -35.6036)
  line L237 (28.3331, -35.6036) -> (28.8968, -35.1476)
  line L238 (28.8968, -35.1476) -> (28.3331, -35.6036)
  arc A237 (29.0658, -33.5479) -> (28.9265, -34.8663) centre (29.6554, -34.2767) ccw
  arc A238 (28.0519, -35.5739) -> (26.7334, -35.4346) centre (27.323, -36.1634) ccw
  line L239 (28.8968, -35.1476) -> (28.3331, -35.6036)
  arc A239 (28.8968, -35.1476) -> (28.9265, -34.8663) centre (28.771, -34.9921) ccw
  arc A240 (28.0519, -35.5739) -> (28.3331, -35.6036) centre (28.2074, -35.4481) ccw
  line L240 (30.8448, -33.4492) -> (30.5783, -33.6949)
  line L241 (30.5783, -33.6949) -> (31.1113, -33.2034)
  line L242 (31.1113, -33.2034) -> (30.5783, -33.6949)
  arc A241 (31.1764, -31.5961) -> (31.1228, -32.9208) centre (31.812, -32.2853) ccw
  arc A242 (30.2957, -33.6835) -> (28.971, -33.6298) centre (29.6065, -34.319) ccw
  line L243 (31.1113, -33.2034) -> (30.5783, -33.6949)
  arc A243 (31.1113, -33.2034) -> (31.1228, -32.9208) centre (30.9757, -33.0564) ccw
  arc A244 (30.2957, -33.6835) -> (30.5783, -33.6949) centre (30.4428, -33.5479) ccw
  line L244 (32.9453, -31.3824) -> (32.6953, -31.6449)
  line L245 (32.6953, -31.6449) -> (33.1953, -31.12)
  line L246 (33.1953, -31.12) -> (32.6953, -31.6449)
  arc A245 (33.1563, -29.5118) -> (33.1885, -30.8372) centre (33.8351, -30.1584) ccw
  arc A246 (32.4125, -31.6518) -> (31.0871, -31.684) centre (31.7659, -32.3306) ccw
  line L247 (33.1953, -31.12) -> (32.6953, -31.6449)
  arc A247 (33.1953, -31.12) -> (33.1885, -30.8372) centre (33.0505, -30.982) ccw
  arc A248 (32.4125, -31.6518) -> (32.6953, -31.6449) centre (32.5505, -31.507) ccw
  line L248 (34.9076, -29.1841) -> (34.6751, -29.4622)
  line L249 (34.6751, -29.4622) -> (35.1401, -28.906)
  line L250 (35.1401, -28.906) -> (34.6751, -29.4622)
  arc A249 (34.997, -27.3037) -> (35.1149, -28.6242) centre (35.7163, -27.905) ccw
  arc A250 (34.3934, -29.4873) -> (33.0728, -29.6053) centre (33.792, -30.2066) ccw
  line L251 (35.1401, -28.906) -> (34.6751, -29.4622)
  arc A251 (35.1401, -28.906) -> (35.1149, -28.6242) centre (34.9867, -28.7777) ccw
  arc A252 (34.3934, -29.4873) -> (34.6751, -29.4622) centre (34.5216, -29.3339) ccw
  line L252 (36.7235, -26.8633) -> (36.5094, -27.1559)
  line L253 (36.5094, -27.1559) -> (36.9375, -26.5707)
  line L254 (36.9375, -26.5707) -> (36.5094, -27.1559)
  arc A253 (36.691, -24.9811) -> (36.8941, -26.2912) centre (37.4476, -25.5346) ccw
  arc A254 (36.2299, -27.1992) -> (34.9198, -27.4024) centre (35.6764, -27.9559) ccw
  line L255 (36.9375, -26.5707) -> (36.5094, -27.1559)
  arc A255 (36.9375, -26.5707) -> (36.8941, -26.2912) centre (36.7761, -26.4527) ccw
  arc A256 (36.2299, -27.1992) -> (36.5094, -27.1559) centre (36.348, -27.0378) ccw
  line L256 (38.3853, -24.4299) -> (38.1907, -24.7357)
  line L257 (38.1907, -24.7357) -> (38.5799, -24.1241)
  line L258 (38.5799, -24.1241) -> (38.1907, -24.7357)
  arc A257 (38.2311, -22.5537) -> (38.5186, -23.8479) centre (39.022, -23.057) ccw
  arc A258 (37.9146, -24.797) -> (36.6203, -25.0846) centre (37.4112, -25.5879) ccw
  line L259 (38.5799, -24.1241) -> (38.1907, -24.7357)
  arc A259 (38.5799, -24.1241) -> (38.5186, -23.8479) centre (38.4112, -24.0167) ccw
  arc A260 (37.9146, -24.797) -> (38.1907, -24.7357) centre (38.0219, -24.6283) ccw
  line L260 (39.8861, -21.894) -> (39.7117, -22.2117)
  line L261 (39.7117, -22.2117) -> (40.0606, -21.5762)
  line L262 (40.0606, -21.5762) -> (39.7117, -22.2117)
  arc A261 (39.6108, -20.0317) -> (39.9815, -21.3046) centre (40.4326, -20.4828) ccw
  arc A262 (39.4402, -22.2908) -> (38.1672, -22.6615) centre (38.989, -23.1127) ccw
  line L263 (40.0606, -21.5762) -> (39.7117, -22.2117)
  arc A263 (40.0606, -21.5762) -> (39.9815, -21.3046) centre (39.8853, -21.4799) ccw
  arc A264 (39.4402, -22.2908) -> (39.7117, -22.2117) centre (39.5364, -22.1155) ccw
  line L264 (41.2197, -19.2662) -> (41.0662, -19.5946)
  line L265 (41.0662, -19.5946) -> (41.3732, -18.9378)
  line L266 (41.3732, -18.9378) -> (41.0662, -19.5946)
  arc A265 (40.8243, -17.4257) -> (41.2767, -18.672) centre (41.6737, -17.8226) ccw
  arc A266 (40.8003, -19.6911) -> (39.554, -20.1435) centre (40.4034, -20.5404) ccw
  line L267 (41.3732, -18.9378) -> (41.0662, -19.5946)
  arc A267 (41.3732, -18.9378) -> (41.2767, -18.672) centre (41.192, -18.8531) ccw
  arc A268 (40.8003, -19.6911) -> (41.0662, -19.5946) centre (40.885, -19.5099) ccw
  line L268 (42.3803, -16.5577) -> (42.2484, -16.8953)
  line L269 (42.2484, -16.8953) -> (42.5123, -16.22)
  line L270 (42.5123, -16.22) -> (42.2484, -16.8953)
  arc A269 (41.8667, -14.7466) -> (42.3988, -15.961) centre (42.7399, -15.0877) ccw
  arc A270 (41.9894, -17.0088) -> (40.775, -17.5409) centre (41.6482, -17.882) ccw
  line L271 (42.5123, -16.22) -> (42.2484, -16.8953)
  arc A271 (42.5123, -16.22) -> (42.3988, -15.961) centre (42.326, -16.1472) ccw
  arc A272 (41.9894, -17.0088) -> (42.2484, -16.8953) centre (42.0621, -16.8225) ccw
  line L272 (43.3632, -13.7797) -> (43.2535, -14.1252)
  line L273 (43.2535, -14.1252) -> (43.473, -13.4342)
  line L274 (43.473, -13.4342) -> (43.2535, -14.1252)
  arc A273 (42.7334, -12.0056) -> (43.343, -13.183) centre (43.6269, -12.2896) ccw
  arc A274 (43.0023, -14.2552) -> (41.8249, -14.8647) centre (42.7184, -15.1487) ccw
  line L275 (43.473, -13.4342) -> (43.2535, -14.1252)
  arc A275 (43.473, -13.4342) -> (43.343, -13.183) centre (43.2824, -13.3736) ccw
  arc A276 (43.0023, -14.2552) -> (43.2535, -14.1252) centre (43.0628, -14.0646) ccw
  line L276 (44.1643, -10.9439) -> (44.0771, -11.2957)
  line L277 (44.0771, -11.2957) -> (44.2514, -10.592)
  line L278 (44.2514, -10.592) -> (44.0771, -11.2957)
  arc A277 (43.4209, -9.2143) -> (44.1054, -10.3498) centre (44.3309, -9.4398) ccw
  arc A278 (43.8348, -11.4418) -> (42.6994, -12.1263) centre (43.6093, -12.3517) ccw
  line L279 (44.2514, -10.592) -> (44.0771, -11.2957)
  arc A279 (44.2514, -10.592) -> (44.1054, -10.3498) centre (44.0573, -10.5439) ccw
  arc A280 (43.8348, -11.4418) -> (44.0771, -11.2957) centre (43.8829, -11.2476) ccw
  line L280 (44.78, -8.0622) -> (44.7158, -8.419)
  line L281 (44.7158, -8.419) -> (44.8443, -7.7054)
  line L282 (44.8443, -7.7054) -> (44.7158, -8.419)
  arc A281 (43.9263, -6.3844) -> (44.6829, -7.4732) centre (44.849, -6.5505) ccw
  arc A282 (44.4835, -8.5804) -> (43.3947, -9.3369) centre (44.3174, -9.503) ccw
  line L283 (44.8443, -7.7054) -> (44.7158, -8.419)
  arc A283 (44.8443, -7.7054) -> (44.6829, -7.4732) centre (44.6474, -7.67) ccw
  arc A284 (44.4835, -8.5804) -> (44.7158, -8.419) centre (44.519, -8.3835) ccw
  line L284 (45.208, -5.1467) -> (45.167, -5.5069)
  line L285 (45.167, -5.5069) -> (45.249, -4.7865)
  line L286 (45.249, -4.7865) -> (45.167, -5.5069)
  arc A285 (44.2475, -3.5276) -> (45.0729, -4.5652) centre (45.1789, -3.6337) ccw
  arc A286 (44.9456, -5.6829) -> (43.9081, -6.5084) centre (44.8396, -6.6144) ccw
  line L287 (45.249, -4.7865) -> (45.167, -5.5069)
  arc A287 (45.249, -4.7865) -> (45.0729, -4.5652) centre (45.0503, -4.7639) ccw
  arc A288 (44.9456, -5.6829) -> (45.167, -5.5069) centre (44.9683, -5.4842) ccw
  line L288 (45.4463, -2.2096) -> (45.4287, -2.5717)
  line L289 (45.4287, -2.5717) -> (45.4639, -1.8475)
  line L290 (45.4639, -1.8475) -> (45.4287, -2.5717)
  arc A289 (44.383, -0.6561) -> (45.2739, -1.638) centre (45.3194, -0.7016) ccw
  arc A290 (45.2192, -2.7617) -> (44.2373, -3.6526) centre (45.1737, -3.6981) ccw
  line L291 (45.4639, -1.8475) -> (45.4287, -2.5717)
  arc A291 (45.4639, -1.8475) -> (45.2739, -1.638) centre (45.2642, -1.8378) ccw
  arc A292 (45.2192, -2.7617) -> (45.4287, -2.5717) centre (45.2289, -2.5619) ccw
  line L292 (45.494, 0.7368) -> (45.4999, 0.3743)
  line L293 (45.4999, 0.3743) -> (45.4882, 1.0992)
  line L294 (45.4882, 1.0992) -> (45.4999, 0.3743)
  arc A293 (44.3324, 2.2182) -> (45.285, 1.296) centre (45.2698, 2.2333) ccw
  arc A294 (45.3032, 0.1711) -> (44.381, -0.7814) centre (45.3184, -0.7663) ccw
  line L295 (45.4882, 1.0992) -> (45.4999, 0.3743)
  arc A295 (45.4882, 1.0992) -> (45.285, 1.296) centre (45.2882, 1.096) ccw
  arc A296 (45.3032, 0.1711) -> (45.4999, 0.3743) centre (45.2999, 0.3711) ccw
  line L296 (45.3509, 3.6801) -> (45.3803, 3.3187)
  line L297 (45.3803, 3.3187) -> (45.3216, 4.0414)
  line L298 (45.3216, 4.0414) -> (45.3803, 3.3187)
  arc A297 (44.0958, 5.0831) -> (45.1061, 4.2245) centre (45.0303, 5.159) ccw
  arc A298 (45.1971, 3.1032) -> (44.3385, 2.093) centre (45.2729, 2.1688) ccw
  line L299 (45.3216, 4.0414) -> (45.3803, 3.3187)
  arc A299 (45.3216, 4.0414) -> (45.1061, 4.2245) centre (45.1223, 4.0252) ccw
  arc A300 (45.1971, 3.1032) -> (45.3803, 3.3187) centre (45.1809, 3.3026) ccw
  line L300 (45.0176, 6.6079) -> (45.0703, 6.2492)
  line L301 (45.0703, 6.2492) -> (44.965, 6.9666)
  line L302 (44.965, 6.9666) -> (45.0703, 6.2492)
  arc A301 (43.6743, 7.9268) -> (44.738, 7.1354) centre (44.6019, 8.063) ccw
  arc A302 (44.9014, 6.0223) -> (44.11, 4.9586) centre (45.0376, 5.0948) ccw
  line L303 (44.965, 6.9666) -> (45.0703, 6.2492)
  arc A303 (44.965, 6.9666) -> (44.738, 7.1354) centre (44.7671, 6.9375) ccw
  arc A304 (44.9014, 6.0223) -> (45.0703, 6.2492) centre (44.8724, 6.2202) ccw
  line L304 (44.4955, 9.508) -> (44.5712, 9.1535)
  line L305 (44.5712, 9.1535) -> (44.4197, 9.8625)
  line L306 (44.4197, 9.8625) -> (44.5712, 9.1535)
  arc A305 (43.0696, 10.7372) -> (44.1823, 10.0163) centre (43.9864, 10.9331) ccw
  arc A306 (44.4174, 8.9161) -> (43.6965, 7.8034) centre (44.6133, 7.9993) ccw
  line L307 (44.4197, 9.8625) -> (44.5712, 9.1535)
  arc A307 (44.4197, 9.8625) -> (44.1823, 10.0163) centre (44.2241, 9.8207) ccw
  arc A308 (44.4174, 8.9161) -> (44.5712, 9.1535) centre (44.3756, 9.1117) ccw
  line L308 (43.7867, 12.3683) -> (43.8852, 12.0194)
  line L309 (43.8852, 12.0194) -> (43.6882, 12.7171)
  line L310 (43.6882, 12.7171) -> (43.8852, 12.0194)
  arc A309 (42.2843, 13.5026) -> (43.4413, 12.8552) centre (43.1865, 13.7574) ccw
  arc A310 (43.7471, 11.7726) -> (43.0998, 10.6155) centre (44.002, 10.8704) ccw
  line L311 (43.6882, 12.7171) -> (43.8852, 12.0194)
  arc A311 (43.6882, 12.7171) -> (43.4413, 12.8552) centre (43.4957, 12.6628) ccw
  arc A312 (43.7471, 11.7726) -> (43.8852, 12.0194) centre (43.6928, 11.9651) ccw
  line L312 (42.8943, 15.1766) -> (43.0152, 14.8349)
  line L313 (43.0152, 14.8349) -> (42.7734, 15.5184)
  line L314 (42.7734, 15.5184) -> (43.0152, 14.8349)
  arc A313 (41.3216, 16.2113) -> (42.5181, 15.6402) centre (42.2054, 16.524) ccw
  arc A314 (42.8934, 14.5796) -> (42.3223, 13.3831) centre (43.2061, 13.6958) ccw
  line L315 (42.7734, 15.5184) -> (43.0152, 14.8349)
  arc A315 (42.7734, 15.5184) -> (42.5181, 15.6402) centre (42.5848, 15.4517) ccw
  arc A316 (42.8934, 14.5796) -> (43.0152, 14.8349) centre (42.8267, 14.7682) ccw
  line L316 (41.8219, 17.9213) -> (41.9647, 17.5882)
  line L317 (41.9647, 17.5882) -> (41.6792, 18.2545)
  line L318 (41.6792, 18.2545) -> (41.9647, 17.5882)
  arc A317 (40.1856, 18.8521) -> (41.4166, 18.3596) centre (41.0473, 19.2213) ccw
  arc A318 (41.8597, 17.3255) -> (41.3672, 16.0946) centre (42.2289, 16.4638) ccw
  line L319 (41.6792, 18.2545) -> (41.9647, 17.5882)
  arc A319 (41.6792, 18.2545) -> (41.4166, 18.3596) centre (41.4953, 18.1758) ccw
  arc A320 (41.8597, 17.3255) -> (41.9647, 17.5882) centre (41.7809, 17.5094) ccw
  line L320 (40.5742, 20.5909) -> (40.7382, 20.2676)
  line L321 (40.7382, 20.2676) -> (40.4101, 20.9141)
  line L322 (40.4101, 20.9141) -> (40.7382, 20.2676)
  arc A321 (38.881, 21.4137) -> (40.1413, 21.002) centre (39.717, 21.838) ccw
  arc A322 (40.6504, 19.9988) -> (40.2387, 18.7385) centre (41.0747, 19.1628) ccw
  line L323 (40.4101, 20.9141) -> (40.7382, 20.2676)
  arc A323 (40.4101, 20.9141) -> (40.1413, 21.002) centre (40.2318, 20.8236) ccw
  arc A324 (40.6504, 19.9988) -> (40.7382, 20.2676) centre (40.5599, 20.1771) ccw
  line L324 (39.1563, 23.1741) -> (39.3409, 22.8621)
  line L325 (39.3409, 22.8621) -> (38.9716, 23.486)
  line L326 (38.9716, 23.486) -> (39.3409, 22.8621)
  arc A325 (37.4134, 23.8856) -> (38.6977, 23.5563) centre (38.2202, 24.3631) ccw
  arc A326 (39.2706, 22.5881) -> (38.9413, 21.3039) centre (39.7481, 21.7813) ccw
  line L327 (38.9716, 23.486) -> (39.3409, 22.8621)
  arc A327 (38.9716, 23.486) -> (38.6977, 23.5563) centre (38.7995, 23.3842) ccw
  arc A328 (39.2706, 22.5881) -> (39.3409, 22.8621) centre (39.1688, 22.7602) ccw
  line L328 (37.5741, 25.66) -> (37.7785, 25.3607)
  line L329 (37.7785, 25.3607) -> (37.3697, 25.9594)
  line L330 (37.3697, 25.9594) -> (37.7785, 25.3607)
  arc A329 (35.7888, 26.2572) -> (37.0917, 26.0118) centre (36.563, 26.786) ccw
  arc A330 (37.7262, 25.0827) -> (37.4807, 23.7798) centre (38.2549, 24.3085) ccw
  line L331 (37.3697, 25.9594) -> (37.7785, 25.3607)
  arc A331 (37.3697, 25.9594) -> (37.0917, 26.0118) centre (37.2045, 25.8466) ccw
  arc A332 (37.7262, 25.0827) -> (37.7785, 25.3607) centre (37.6134, 25.2479) ccw
  line L332 (35.8343, 28.0384) -> (36.0577, 27.7529)
  line L333 (36.0577, 27.7529) -> (35.6109, 28.3239)
  line L334 (35.6109, 28.3239) -> (36.0577, 27.7529)
  arc A333 (34.0141, 28.5188) -> (35.3302, 28.3582) centre (34.7525, 29.0965) ccw
  arc A334 (36.0234, 27.4721) -> (35.8628, 26.1561) centre (36.6011, 26.7338) ccw
  line L335 (35.6109, 28.3239) -> (36.0577, 27.7529)
  arc A335 (35.6109, 28.3239) -> (35.3302, 28.3582) centre (35.4534, 28.2006) ccw
  arc A336 (36.0234, 27.4721) -> (36.0577, 27.7529) centre (35.9002, 27.6297) ccw
  line L336 (33.9442, 30.2991) -> (34.1856, 30.0287)
  line L337 (34.1856, 30.0287) -> (33.7029, 30.5696)
  line L338 (33.7029, 30.5696) -> (34.1856, 30.0287)
  arc A337 (32.0968, 30.6607) -> (33.4205, 30.5856) centre (32.7962, 31.285) ccw
  arc A338 (34.1696, 29.7463) -> (34.0945, 28.4226) centre (34.7939, 29.0469) ccw
  line L339 (33.7029, 30.5696) -> (34.1856, 30.0287)
  arc A339 (33.7029, 30.5696) -> (33.4205, 30.5856) centre (33.5536, 30.4364) ccw
  arc A340 (34.1696, 29.7463) -> (34.1856, 30.0287) centre (34.0364, 29.8955) ccw
  line L340 (31.9118, 32.4328) -> (32.1702, 32.1786)
  line L341 (32.1702, 32.1786) -> (31.6534, 32.687)
  line L342 (31.6534, 32.687) -> (32.1702, 32.1786)
  arc A341 (30.0448, 32.674) -> (31.3706, 32.6848) centre (30.7023, 33.3423) ccw
  arc A342 (32.1725, 31.8957) -> (32.1832, 30.5699) centre (32.8407, 31.2382) ccw
  line L343 (31.6534, 32.687) -> (32.1702, 32.1786)
  arc A343 (31.6534, 32.687) -> (31.3706, 32.6848) centre (31.5131, 32.5445) ccw
  arc A344 (32.1725, 31.8957) -> (32.1702, 32.1786) centre (32.0299, 32.036) ccw
  line L344 (29.7455, 34.4304) -> (30.0198, 34.1934)
  line L345 (30.0198, 34.1934) -> (29.4712, 34.6674)
  line L346 (29.4712, 34.6674) -> (30.0198, 34.1934)
  arc A345 (27.8668, 34.5503) -> (29.1891, 34.6468) centre (28.4797, 35.2597) ccw
  arc A346 (30.0404, 33.9114) -> (30.1369, 32.5891) centre (30.7498, 33.2985) ccw
  line L347 (29.4712, 34.6674) -> (30.0198, 34.1934)
  arc A347 (29.4712, 34.6674) -> (29.1891, 34.6468) centre (29.3405, 34.5161) ccw
  arc A348 (30.0404, 33.9114) -> (30.0198, 34.1934) centre (29.8891, 34.0421) ccw
  line L348 (27.4545, 36.2836) -> (27.7435, 36.0649)
  line L349 (27.7435, 36.0649) -> (27.1654, 36.5024)
  line L350 (27.1654, 36.5024) -> (27.7435, 36.0649)
  arc A349 (25.5719, 36.2816) -> (26.8852, 36.4636) centre (26.1376, 37.0293) ccw
  arc A350 (27.7823, 35.7847) -> (27.9643, 34.4715) centre (28.5299, 35.2191) ccw
  line L351 (27.1654, 36.5024) -> (27.7435, 36.0649)
  arc A351 (27.1654, 36.5024) -> (26.8852, 36.4636) centre (27.0447, 36.3429) ccw
  arc A352 (27.7823, 35.7847) -> (27.7435, 36.0649) centre (27.6228, 35.9054) ccw
  line L352 (25.0482, 37.9847) -> (25.3509, 37.7851)
  line L353 (25.3509, 37.7851) -> (24.7456, 38.1842)
  line L354 (24.7456, 38.1842) -> (25.3509, 37.7851)
  arc A353 (23.1698, 37.8608) -> (24.4685, 38.1274) centre (23.6859, 38.6435) ccw
  arc A354 (25.4077, 37.508) -> (25.6743, 36.2093) centre (26.1904, 36.9919) ccw
  line L355 (24.7456, 38.1842) -> (25.3509, 37.7851)
  arc A355 (24.7456, 38.1842) -> (24.4685, 38.1274) centre (24.6355, 38.0173) ccw
  arc A356 (25.4077, 37.508) -> (25.3509, 37.7851) centre (25.2408, 37.6182) ccw
  line L356 (22.537, 39.5264) -> (22.8519, 39.3468)
  line L357 (22.8519, 39.3468) -> (22.2221, 39.7059)
  line L358 (22.2221, 39.7059) -> (22.8519, 39.3468)